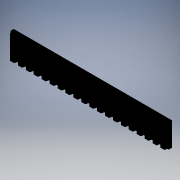
# Autodesk Inventor part: HTBOG-S5M150-366
Saved by Autodesk Inventor 2017.3 (Build 213256000, 256)
## iProperties
Part Number: HTBOG-S5M150-366
Material: Generic
Catalog Web Link: www.cadenas.de
Description: HTBO-S3M, HTBO-S5M, HTBO-S8M, HTBOG-S5M, HTBOG-S8M-Open End Belts - S Type
Vendor: MISUMI
Document SubType Name: Modeling
Designer: partserver
Manufacturer: MISUMI
Mass: 4.42324 g
Surface Area: 44.5783 cm^2
Volume: 4.42324 cm^3
Density: 1 g/cm^3
Appearance: PSOLRGB-0-0-0
Category: PARTsolutions
Company: MISUMI
Title: HTBOG-S5M150-366
Author: Cadenas PARTsolutions
Comments: Open End Belts - S Type
PSOL_IDENT_0: {$CADENAS_DATA\23d-libs\misumi\metric\48_timing_belts\htbog_s5m.prj},230 {VTYP=3D},{NB=HTBOG-S5M150-
PSOL_IDENT_1: 366},{LINA=HTBOG-S5M150-366},{NN=HTBO-S3M, HTBO-S5M, HTBO-S8M, HTBOG-S5M, HTBOG-S8M},{DATE=30.06.202
PSOL_IDENT_2: 1 13:24:08},{GEOMDATE=28.08.2009 09:14:00},{VERSION=},{LINEID=40},{WBVAR=MATMB,BNW,NT},{WBNUMERIC=NT
PSOL_IDENT_3: }  {NB=HTBOG-S5M150-366},{LINA=HTBOG-S5M150-366},{KT=DUMMY},{PN=HTBOG-S5M150-366},{MATMB=G},{MATMBAL
PSOL_IDENT_4: G=  'G','Chloroprene Rubber','','Polyurethane'                       },{MATCW=Glass Cord},{COLOR=Bla
PSOL_IDENT_5: ck},{OT=-20~80},{TB=S5M},{BNW=150},{NT=366},{BW=15},{AT=490},{MAX=20},{AMJ=TBCK-S5M150},{PITCH=5},{R
PSOL_IDENT_6: AA=3.25},{LRR=3.25},{H=3.60},{HH=1.91},{II=2.00},{PLD=0.480},{UM=38.8},{BNWALG= '100','100','150','1
PSOL_IDENT_7: 50'},{NTALG=[50:4000]},{NOTE=3D Model is Only a Segment of the Actual Belt},{COL=0.00,0.00,0.00,0.00
PSOL_IDENT_8: }
NB: HTBOG-S5M150-366
NN: HTBO-S3M, HTBO-S5M, HTBO-S8M, HTBOG-S5M, HTBOG-S8M
NT: 366
NBSYN: $PN.
LINA: HTBOG-S5M150-366
CATALOG: Misumi
PN: HTBOG-S5M150-366
MATMB: Chloroprene Rubber
MATCW: Glass Cord
COLOR: Black
OT: -20~80
TB: S5M
BNW: 150
BW: 15
AT: 490
AMJ: TBCK-S5M150
PITCH: 5
RAA: 3.25
LRR: 3.25
H: 3.6
HH: 1.91
II: 2
PLD: 0.48
UM: 38.8
NOTE: 3D Model is Only a Segment of the Actual Belt
SUPPLIER: MISUMI
ARTICLENO: HTBOG-S5M150-366
BOMINFO: HTBOG-S5M150-366
CREATOR: CADENAS GmbH
Autodesk Inventor part; units mm, degrees
ref_plane "YZ Plane" through (0, 0, 0) normal (1, 0, 0) x (0, 1, 0)
ref_plane "XZ Plane" through (0, 0, 0) normal (0, 1, 0) x (-1, 0, 0)
ref_plane "XY Plane" through (0, 0, 0) normal (0, 0, 1) x (1, 0, 0)
sketch "Sketch_1" plane through (0, 0, 0) normal (0, 0, 1) x (1, 0, 0)
  line L0 (-5, -1) -> (-4.125, -1)
  arc A0 (-4.125, -1) -> (-3.7039, -2.6) centre (-0.875, -1) ccw
  line L1 (-3.7039, -2.6) -> (-1.2961, -2.6)
  arc A1 (-1.2961, -2.6) -> (-0.875, -1) centre (-4.125, -1) ccw
  line L2 (-0.875, -1) -> (-0.1, -1)
  line L3 (-0.1, -1) -> (-0.1, -0.9)
  line L4 (-0.1, -0.9) -> (0.1, -0.9)
  line L5 (0.1, -0.9) -> (0.1, -1)
  line L6 (0.1, -1) -> (0.875, -1)
  arc A2 (0.875, -1) -> (1.2961, -2.6) centre (4.125, -1) ccw
  line L7 (1.2961, -2.6) -> (3.7039, -2.6)
  arc A3 (3.7039, -2.6) -> (4.125, -1) centre (0.875, -1) ccw
  line L8 (4.125, -1) -> (4.9, -1)
  line L9 (4.9, -1) -> (4.9, -0.9)
  line L10 (4.9, -0.9) -> (5.1, -0.9)
  line L11 (5.1, -0.9) -> (5.1, -1)
  line L12 (5.1, -1) -> (5.875, -1)
  arc A4 (5.875, -1) -> (6.2961, -2.6) centre (9.125, -1) ccw
  line L13 (6.2961, -2.6) -> (8.7039, -2.6)
  arc A5 (8.7039, -2.6) -> (9.125, -1) centre (5.875, -1) ccw
  line L14 (9.125, -1) -> (9.9, -1)
  line L15 (9.9, -1) -> (9.9, -0.9)
  line L16 (9.9, -0.9) -> (10.1, -0.9)
  line L17 (10.1, -0.9) -> (10.1, -1)
  line L18 (10.1, -1) -> (10.875, -1)
  arc A6 (10.875, -1) -> (11.2961, -2.6) centre (14.125, -1) ccw
  line L19 (11.2961, -2.6) -> (13.7039, -2.6)
  arc A7 (13.7039, -2.6) -> (14.125, -1) centre (10.875, -1) ccw
  line L20 (14.125, -1) -> (14.9, -1)
  line L21 (14.9, -1) -> (14.9, -0.9)
  line L22 (14.9, -0.9) -> (15.1, -0.9)
  line L23 (15.1, -0.9) -> (15.1, -1)
  line L24 (15.1, -1) -> (15.875, -1)
  arc A8 (15.875, -1) -> (16.2961, -2.6) centre (19.125, -1) ccw
  line L25 (16.2961, -2.6) -> (18.7039, -2.6)
  arc A9 (18.7039, -2.6) -> (19.125, -1) centre (15.875, -1) ccw
  line L26 (19.125, -1) -> (19.9, -1)
  line L27 (19.9, -1) -> (19.9, -0.9)
  line L28 (19.9, -0.9) -> (20.1, -0.9)
  line L29 (20.1, -0.9) -> (20.1, -1)
  line L30 (20.1, -1) -> (20.875, -1)
  arc A10 (20.875, -1) -> (21.2961, -2.6) centre (24.125, -1) ccw
  line L31 (21.2961, -2.6) -> (23.7039, -2.6)
  arc A11 (23.7039, -2.6) -> (24.125, -1) centre (20.875, -1) ccw
  line L32 (24.125, -1) -> (24.9, -1)
  line L33 (24.9, -1) -> (24.9, -0.9)
  line L34 (24.9, -0.9) -> (25.1, -0.9)
  line L35 (25.1, -0.9) -> (25.1, -1)
  line L36 (25.1, -1) -> (25.875, -1)
  arc A12 (25.875, -1) -> (26.2961, -2.6) centre (29.125, -1) ccw
  line L37 (26.2961, -2.6) -> (28.7039, -2.6)
  arc A13 (28.7039, -2.6) -> (29.125, -1) centre (25.875, -1) ccw
  line L38 (29.125, -1) -> (29.9, -1)
  line L39 (29.9, -1) -> (29.9, -0.9)
  line L40 (29.9, -0.9) -> (30.1, -0.9)
  line L41 (30.1, -0.9) -> (30.1, -1)
  line L42 (30.1, -1) -> (30.875, -1)
  arc A14 (30.875, -1) -> (31.2961, -2.6) centre (34.125, -1) ccw
  line L43 (31.2961, -2.6) -> (33.7039, -2.6)
  arc A15 (33.7039, -2.6) -> (34.125, -1) centre (30.875, -1) ccw
  line L44 (34.125, -1) -> (34.9, -1)
  line L45 (34.9, -1) -> (34.9, -0.9)
  line L46 (34.9, -0.9) -> (35.1, -0.9)
  line L47 (35.1, -0.9) -> (35.1, -1)
  line L48 (35.1, -1) -> (35.875, -1)
  arc A16 (35.875, -1) -> (36.2961, -2.6) centre (39.125, -1) ccw
  line L49 (36.2961, -2.6) -> (38.7039, -2.6)
  arc A17 (38.7039, -2.6) -> (39.125, -1) centre (35.875, -1) ccw
  line L50 (39.125, -1) -> (39.9, -1)
  line L51 (39.9, -1) -> (39.9, -0.9)
  line L52 (39.9, -0.9) -> (40.1, -0.9)
  line L53 (40.1, -0.9) -> (40.1, -1)
  line L54 (40.1, -1) -> (40.875, -1)
  arc A18 (40.875, -1) -> (41.2961, -2.6) centre (44.125, -1) ccw
  line L55 (41.2961, -2.6) -> (43.7039, -2.6)
  arc A19 (43.7039, -2.6) -> (44.125, -1) centre (40.875, -1) ccw
  line L56 (44.125, -1) -> (44.9, -1)
  line L57 (44.9, -1) -> (44.9, -0.9)
  line L58 (44.9, -0.9) -> (45.1, -0.9)
  line L59 (45.1, -0.9) -> (45.1, -1)
  line L60 (45.1, -1) -> (45.875, -1)
  arc A20 (45.875, -1) -> (46.2961, -2.6) centre (49.125, -1) ccw
  line L61 (46.2961, -2.6) -> (48.7039, -2.6)
  arc A21 (48.7039, -2.6) -> (49.125, -1) centre (45.875, -1) ccw
  line L62 (49.125, -1) -> (49.9, -1)
  line L63 (49.9, -1) -> (49.9, -0.9)
  line L64 (49.9, -0.9) -> (50.1, -0.9)
  line L65 (50.1, -0.9) -> (50.1, -1)
  line L66 (50.1, -1) -> (50.875, -1)
  arc A22 (50.875, -1) -> (51.2961, -2.6) centre (54.125, -1) ccw
  line L67 (51.2961, -2.6) -> (53.7039, -2.6)
  arc A23 (53.7039, -2.6) -> (54.125, -1) centre (50.875, -1) ccw
  line L68 (54.125, -1) -> (54.9, -1)
  line L69 (54.9, -1) -> (54.9, -0.9)
  line L70 (54.9, -0.9) -> (55.1, -0.9)
  line L71 (55.1, -0.9) -> (55.1, -1)
  line L72 (55.1, -1) -> (55.875, -1)
  arc A24 (55.875, -1) -> (56.2961, -2.6) centre (59.125, -1) ccw
  line L73 (56.2961, -2.6) -> (58.7039, -2.6)
  arc A25 (58.7039, -2.6) -> (59.125, -1) centre (55.875, -1) ccw
  line L74 (59.125, -1) -> (59.9, -1)
  line L75 (59.9, -1) -> (59.9, -0.9)
  line L76 (59.9, -0.9) -> (60.1, -0.9)
  line L77 (60.1, -0.9) -> (60.1, -1)
  line L78 (60.1, -1) -> (60.875, -1)
  arc A26 (60.875, -1) -> (61.2961, -2.6) centre (64.125, -1) ccw
  line L79 (61.2961, -2.6) -> (63.7039, -2.6)
  arc A27 (63.7039, -2.6) -> (64.125, -1) centre (60.875, -1) ccw
  line L80 (64.125, -1) -> (64.9, -1)
  line L81 (64.9, -1) -> (64.9, -0.9)
  line L82 (64.9, -0.9) -> (65.1, -0.9)
  line L83 (65.1, -0.9) -> (65.1, -1)
  line L84 (65.1, -1) -> (65.875, -1)
  arc A28 (65.875, -1) -> (66.2961, -2.6) centre (69.125, -1) ccw
  line L85 (66.2961, -2.6) -> (68.7039, -2.6)
  arc A29 (68.7039, -2.6) -> (69.125, -1) centre (65.875, -1) ccw
  line L86 (69.125, -1) -> (69.9, -1)
  line L87 (69.9, -1) -> (69.9, -0.9)
  line L88 (69.9, -0.9) -> (70.1, -0.9)
  line L89 (70.1, -0.9) -> (70.1, -1)
  line L90 (70.1, -1) -> (70.875, -1)
  arc A30 (70.875, -1) -> (71.2961, -2.6) centre (74.125, -1) ccw
  line L91 (71.2961, -2.6) -> (73.7039, -2.6)
  arc A31 (73.7039, -2.6) -> (74.125, -1) centre (70.875, -1) ccw
  line L92 (74.125, -1) -> (74.9, -1)
  line L93 (74.9, -1) -> (74.9, -0.9)
  line L94 (74.9, -0.9) -> (75.1, -0.9)
  line L95 (75.1, -0.9) -> (75.1, -1)
  line L96 (75.1, -1) -> (75.875, -1)
  arc A32 (75.875, -1) -> (76.2961, -2.6) centre (79.125, -1) ccw
  line L97 (76.2961, -2.6) -> (78.7039, -2.6)
  arc A33 (78.7039, -2.6) -> (79.125, -1) centre (75.875, -1) ccw
  line L98 (79.125, -1) -> (79.9, -1)
  line L99 (79.9, -1) -> (79.9, -0.9)
  line L100 (79.9, -0.9) -> (80.1, -0.9)
  line L101 (80.1, -0.9) -> (80.1, -1)
  line L102 (80.1, -1) -> (80.875, -1)
  arc A34 (80.875, -1) -> (81.2961, -2.6) centre (84.125, -1) ccw
  line L103 (81.2961, -2.6) -> (83.7039, -2.6)
  arc A35 (83.7039, -2.6) -> (84.125, -1) centre (80.875, -1) ccw
  line L104 (84.125, -1) -> (84.9, -1)
  line L105 (84.9, -1) -> (84.9, -0.9)
  line L106 (84.9, -0.9) -> (85.1, -0.9)
  line L107 (85.1, -0.9) -> (85.1, -1)
  line L108 (85.1, -1) -> (85.875, -1)
  arc A36 (85.875, -1) -> (86.2961, -2.6) centre (89.125, -1) ccw
  line L109 (86.2961, -2.6) -> (88.7039, -2.6)
  arc A37 (88.7039, -2.6) -> (89.125, -1) centre (85.875, -1) ccw
  line L110 (89.125, -1) -> (89.9, -1)
  line L111 (89.9, -1) -> (89.9, -0.9)
  line L112 (89.9, -0.9) -> (90.1, -0.9)
  line L113 (90.1, -0.9) -> (90.1, -1)
  line L114 (90.1, -1) -> (90.875, -1)
  arc A38 (90.875, -1) -> (91.2961, -2.6) centre (94.125, -1) ccw
  line L115 (91.2961, -2.6) -> (93.7039, -2.6)
  arc A39 (93.7039, -2.6) -> (94.125, -1) centre (90.875, -1) ccw
  line L116 (94.125, -1) -> (95, -1)
  line L117 (95, -1) -> (95, 1)
  line L118 (95, 1) -> (-5, 1)
  line L119 (-5, 1) -> (-5, -1)
  constraints: 240 end point, 80 point on circle, 40 centre point
extrude "Extrusion1" add sketch "Sketch_1" along normal mid plane 15
body "Solid1"
